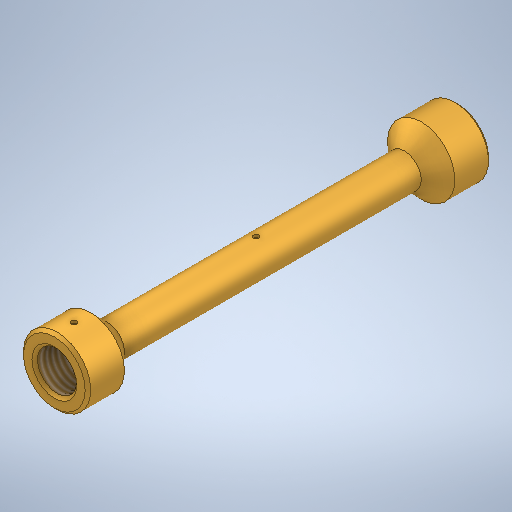
# Autodesk Inventor part: Heater
Saved by Autodesk Inventor 2025.2 (Build 292293000, 293)
## iProperties
Created: 2026-06-11
Part Number: Heater
Material: Generic
Document SubType Name: Modeling
Designer: Simon
Density: 1 g/cm^3
Appearance: Brass - Satin
Author: Simon
Autodesk Inventor part; units mm, degrees
ref_plane "YZ Plane" through (0, 0, 0) normal (1, 0, 0) x (0, 1, 0)
ref_plane "XY Plane" through (0, 0, 0) normal (0, 0, 1) x (1, 0, 0)
sketch "Sketch1" plane through (0, 0, 0) normal (1, 0, 0) x (0, 1, 0)
  line L0 (0, 0) -> (0, -72)
  line L1 (0, -72) -> (3.5, -72)
  line L2 (3.5, -72) -> (3.5, 0)
  line L3 (3.5, 0) -> (0, 0)
  line L4 (3.5, 0) -> (3.5, -6)
  line L5 (3.5, -72) -> (3.5, -66)
  line L6 (3.5, -72) -> (6, -72)
  line L7 (6, -72) -> (6, -66)
  line L8 (6, -66) -> (3.5, -66)
  line L9 (3.5, 0) -> (6, 0)
  line L10 (6, 0) -> (6, -6)
  line L11 (6, -6) -> (3.5, -6)
  line L12 (3.5, -66) -> (1, -66)
  line L13 (1, -66) -> (1, -6)
  line L14 (1, -6) -> (3.5, -6)
  line L15 (6, -6) -> (6, -7)
  line L16 (6, -7) -> (1, -7)
  line L17 (6, -66) -> (6, -65)
  line L18 (6, -65) -> (1, -65)
  line L19 (3.5, -7) -> (3.6267, -7)
  line L20 (3, -7) -> (3, -65)
  point P0 (3.5, -65)
  point P1 (2, -6)
  point P2 (3.6267, -65)
  dimension "d0" = 72
  dimension "d1" = 3.5
  dimension "d2" = 6
  dimension "d3" = 6
  dimension "d5" = 2.5
  dimension "d6" = 2.5
  dimension "d7" = 2.5
  dimension "d8" = 1
  dimension "d9" = 1
  dimension "d22" = 2
  constraints: 42 end point, 12 point on line, 11 perpendicular, 2 vertical, 1 horizontal, 1 midpoint, 1 parallel
  measures "d0" distance of L0.start L0.end
  measures "d1" distance of L0.end L1.end
  measures "d2" distance of L2.end L4.end
  measures "d3" distance of L1.end L5.end
  measures "d5" distance of L1.end L6.end
  measures "d6" distance of L2.end L9.end
  measures "d7" distance of L5.end L12.end
  measures "d8" distance of L10.end L15.end
  measures "d9" distance of L7.end L17.end
  measures "d22" distance between parallel lines of L20 L13
revolve "Revolution1" add sketch "Sketch1" angle 360 about axis through (0, 0, 0) along (0, 0, -1) contours L9 L10 L11 L2 | L2 L8 L7 L6 | L11 L15 L16 L2 | L2 L16 L13 L14 | L12 L13 L18 L2 | L2 L18 L17 L8 | L20 L18 L13 L16
thread "Thread1" size "M7x1" class "6H" standard "ANSI Metric M Profile" full length
thread "Thread2" size "M7x1" class "6H" standard "ANSI Metric M Profile" full length
chamfer "Chamfer1" distance 0.5 angle 45 2 edges at (0, -3.5, 0) (0, -3.5, -72)
chamfer "Chamfer2" distance 0.5 angle 45 4 edges at (0, -6, -72) (0, -6, -65) (0, -6, -7) (0, -6, 0)
chamfer "Chamfer3" distance 2.5 angle 45 2 edges at (0, -3, -7) (0, -3, -65)
ref_plane "Work Plane1" through (0, 6, -3.5) normal (0, 1, 0) x (-1, 0, 0)
ref_plane "Work Plane2" through (0, 3, -36) normal (0, 1, 0) x (-1, 0, 0)
sketch "Sketch2" plane through (0, 6, -3.5) normal (0, 1, 0) x (-1, 0, 0)
  point P0 (0, 3.5)
  point P1 (0, 0)
  point P2 (0, 0)
  constraints: 1 coincident
sketch "Sketch3" plane through (0, 3, -36) normal (0, 1, 0) x (-1, 0, 0)
  point P0 (0, 36)
  point P1 (0, 0)
hole "Hole1" at (0, 6, -3.5) direction (0, -1, 0) diameter 1 depth 0.5 tip angle 118
hole "Hole2" at (0, 3, -36) direction (0, -1, 0) diameter 1 depth 0.5 tip angle 118
body "Solid1"
